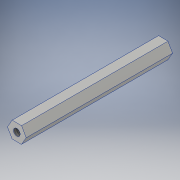
# Autodesk Inventor part: Hex Standoff 6-32 x2250
Saved by Autodesk Inventor 2017 (Build 210142000, 142)
## iProperties
Created: 2018-04-21
Part Number: Hex Standoff 6-32 x2250
Material: Aluminum 6061
Document SubType Name: Modeling
Designer: User
Density: 2.7 g/cm^3
Appearance: Aluminum - Flat
Mass: 4.5427 g
Surface Area: 17.9029 cm^2
Volume: 1.68248 cm^3
Author: User
Autodesk Inventor part; units mm, degrees
ref_plane "YZ Plane" through (0, 0, 0) normal (1, 0, 0) x (0, 1, 0)
ref_plane "XZ Plane" through (0, 0, 0) normal (0, 1, 0) x (-1, 0, 0)
ref_plane "XY Plane" through (0, 0, 0) normal (0, 0, 1) x (1, 0, 0)
sketch "Sketch1" plane through (0, 0, 0) normal (0, 0, 1) x (1, 0, 0)
  line L0 (1.8641, 3.1569) -> (3.666, -0.0359)
  line L1 (3.666, -0.0359) -> (1.8019, -3.1928)
  line L2 (1.8019, -3.1928) -> (-1.8641, -3.1569)
  line L3 (-1.8641, -3.1569) -> (-3.666, 0.0359)
  line L4 (-3.666, 0.0359) -> (-1.8019, 3.1928)
  line L5 (-1.8019, 3.1928) -> (1.8641, 3.1569)
  point P0 (0, 0)
  point P1 (0, 0)
  point P2 (0, 0)
  dimension "d0" = 6.35
  constraints: 12 end point, 2 coincident, 13 other
  measures "d0" distance between parallel lines of L2 L5
extrude "Extrusion1" add sketch "Sketch1" along normal blind 57.15
hole "Hole1" at (0, 0, 0) direction (0, 0, 1) diameter 2.6416 depth 57.15 tip angle 118 thread size "6-32 UNC" class "2B" standard "ANSI Unified Screw Threads"
body "Solid1"
